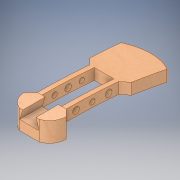
# Autodesk Inventor part: tenjin
Saved by Autodesk Inventor 2019 (Build 230136000, 136)
## iProperties
Created: 2019-11-15
Part Number: tenjin
Material: Клен
Document SubType Name: Modeling
Designer: stepa
Density: 0.705 g/cm^3
Appearance: Клен — массив — натуральный — с умеренным глянцем
Mass: 93.0238 g
Surface Area: 297.423 cm^2
Volume: 131.949 cm^3
Author: stepa
Autodesk Inventor part; units mm, degrees
ref_plane "YZ Plane" through (0, 0, 0) normal (1, 0, 0) x (0, 1, 0)
ref_plane "XZ Plane" through (0, 0, 0) normal (0, 1, 0) x (-1, 0, 0)
ref_plane "XY Plane" through (0, 0, 0) normal (0, 0, 1) x (1, 0, 0)
sketch "Эскиз1" plane through (0, 0, 0) normal (0, 1, 0) x (-1, 0, 0)
  line L0 (15, -40) -> (-15, -40)
  line L1 (-15, -40) -> (-15, 40)
  line L2 (-15, 40) -> (15, 40)
  line L3 (15, 40) -> (15, -40)
  line L4 (22, -40) -> (22, 40)
  line L5 (22, 40) -> (32, 50)
  line L6 (22, -40) -> (32, -50)
  line L7 (-22, -40) -> (-22, 40)
  line L8 (-22, -40) -> (-32, -50)
  line L9 (-22, 40) -> (-32, 50)
  line L10 (-32, -50) -> (-35, -101)
  line L11 (32, -50) -> (35, -101)
  arc A0 (-35, -101) -> (35, -101) centre (0, -44.75) ccw
  line L12 (15, 74) -> (-15, 74)
  arc A1 (32, 50) -> (15, 74) centre (6.5588, 50) ccw
  arc A2 (-15, 74) -> (-32, 50) centre (-6.5588, 50) ccw
  line L13 (32, -50) -> (32, 50)
  line L14 (-32, -50) -> (-32, 50)
  point P0 (0, 0)
  point P1 (0, -40)
  point P2 (0, -111)
  point P3 (15, 0)
  dimension "d0" = 30
  dimension "d1" = 80
  dimension "d2" = 135
  dimension "d3" = 135
  dimension "d6" = 10
  dimension "d7" = 64
  dimension "d8" = 70
  dimension "d9" = 71
  dimension "d10" = 10
  dimension "d11" = 44
  dimension "d12" = 34
  dimension "d13" = 10
  constraints: 30 end point, 7 point on circle, 6 equal length, 5 horizontal alignment, 4 vertical alignment, 3 centre point, 3 vertical, 2 horizontal, 2 midpoint, 2 parallel, 1 perpendicular, 1 point on line, 1 tangent
  measures "d0" distance of L0.start L0.end
  measures "d1" distance of L0.end L1.end
  measures "d2" angle of L6 L4
  measures "d3" angle of L8 L7
  measures "d6" horizontal distance of L4.start L6.end
  measures "d7" distance of L6.end L8.end
  measures "d8" distance of L10.end L11.end
  measures "d9" distance from line of L0 point (0, -111)
  measures "d10" vertical distance of point (0, -111) L10.end
  measures "d11" distance between parallel lines of L7 L4
  measures "d12" distance between parallel lines of L12 L2
  measures "d13" horizontal distance of L5.end L4.end
extrude "Выдавливание1" add sketch "Эскиз1" along normal blind 30 contours L6 L11 A0 L10 L8 L7 L9 A2 L12 A1 L5 L4
ref_plane "РабПлоскость1" through (42, 0, 40) normal (1, 0, 0) x (0, 0, -1)
sketch "Эскиз3" plane through (42, 0, 40) normal (1, 0, 0) x (0, 0, -1)
  line L0 (-10, 0) -> (0, 0) projected
  line L1 (-10, 0) -> (0, 13)
  line L2 (-10, 0) -> (151, 0)
  arc A0 (151, 0) -> (0, 13) centre (0, -870.4615) ccw
  line L3 (80, 30) -> (0, 30) projected
  arc A1 (151, 17.249) -> (0, 30) centre (0, -870.4615) ccw
  line L4 (151, 0) -> (141, 0) projected
  line L5 (151, 0) -> (151, 17.249)
  line L6 (151, 0) -> (151, 30) projected
  line L7 (0, 30) -> (151, 30)
  line L8 (-10, 30) -> (0, 30) projected
  line L9 (0, 0) -> (0, 30) projected
  point P0 (40, 0)
  dimension "d19" = 17
  constraints: 8 end point, 4 point on circle, 2 centre point, 2 horizontal, 1 collinear, 1 concentric, 1 point on line, 1 tangent, 1 vertical alignment
  measures "d19" distance of L3.end L1.end
extrude "Выдавливание2" cut sketch "Эскиз3" against normal through all contours L9 A0 L2 | L3 L7 L6 A1
chamfer "Фаска1" distance 10 distance2 13 1 edges at (0, 0, 40) measured on face at (0, 0, 40.5)
sketch "Эскиз5" plane through (-15, 0, 74) normal (0, 0, 1) x (1, 0, 0)
  line L0 (0, 0) -> (30, 0) projected
  line L1 (30, 0) -> (30, 30) projected
  line L2 (0, 30) -> (30, 30) projected
  line L3 (0, 0) -> (0, 30) projected
  line L4 (5, 30) -> (0, 15)
  line L5 (25, 30) -> (30, 15)
  line L6 (0, 15) -> (30, 15)
  line L7 (5, 30) -> (25, 30)
  point P0 (15, 0)
  dimension "d31" = 15
  dimension "d32" = 20
  constraints: 8 end point, 2 horizontal, 2 midpoint, 2 point on line, 1 equal length, 1 horizontal alignment
  measures "d31" distance between parallel lines of L2 L6
  measures "d32" distance of L5.start L4.start
extrude "Выдавливание3" cut sketch "Эскиз5" against normal up to next contours L4 L2 L5 L6
sketch "Эскиз6" plane through (0, 30, 0) normal (0, 1, 0) x (1, 0, 0)
  line L0 (15, 40) -> (-15, 40) projected
  line L1 (15, -40) -> (15, 40) projected
  line L2 (15, -40) -> (22, -40) projected
  line L3 (22, 40) -> (22, -40) projected
  line L4 (32, 50) -> (22, 40) projected
  line L5 (35, 101) -> (32, 50) projected
  line L6 (-32, 50) -> (-35, 101) projected
  line L7 (18, 0) -> (-32, 50) projected
  line L8 (-22, -40) -> (-22, -40) projected
  line L9 (-22, -40) -> (-15, -40) projected
  line L10 (-15, 40) -> (-15, -40) projected
  line L11 (-22, 0) -> (22, 0)
  line L12 (-22, -40) -> (-22, -40) projected
  line L13 (-22, 20) -> (22, 25)
  line L14 (-22, -20) -> (22, -25)
  point P0 (0, 0)
  dimension "d35" = 20
  dimension "d36" = 20
  dimension "d37" = 25
  dimension "d38" = 25
  constraints: 6 end point, 5 point on line, 1 midpoint, 2 other
  measures "d35" distance of L14.start L11.start
  measures "d36" distance of L13.start L11.start
  measures "d37" distance of L11.end L13.end
  measures "d38" distance of L11.end L14.end
ref_plane "РабПлоскость2" through (-22, 30, 20) normal (-0.1129097, 0, 0.9936053) x (0.9936053, 0, 0.1129097)
ref_plane "РабПлоскость3" through (-22, 30, 0) normal (0, 0, 1) x (1, 0, 0)
ref_plane "РабПлоскость4" through (-22, 30, -20) normal (0.1129097, 0, 0.9936053) x (0.9936053, 0, -0.1129097)
ref_plane "РабПлоскость5" through (22, 21.5, 40) normal (0, -0.9989917, 0.0448943) x (0, -0.0448943, -0.9989917)
hole "Отверстие1" at (22, 20.8259, 25) direction (-0.9935925, -0.0050741, -0.1129082) diameter 10 end up to surface start extended yes
hole "Отверстие2" at (22, 18.5789, -25) direction (0.9935925, -0.0050741, -0.1129082) diameter 10 end up to surface start extended yes
hole "Отверстие3" at (22, 19.7024, 0) direction (-1, 0, 0) diameter 8 depth 7 tip angle 118 start extended yes
hole "Отверстие4" at (-22, 20.6012, 20) direction (0.9935925, 0.0050741, 0.1129082) diameter 8 end up to surface start extended yes
hole "Отверстие5" at (-22, 18.8036, -20) direction (0.9935925, -0.0050741, -0.1129082) diameter 8 end up to surface start extended yes
hole "Отверстие6" at (-22, 19.7024, 0) direction (1, 0, 0) diameter 10 depth 7 tip angle 118 start extended yes
